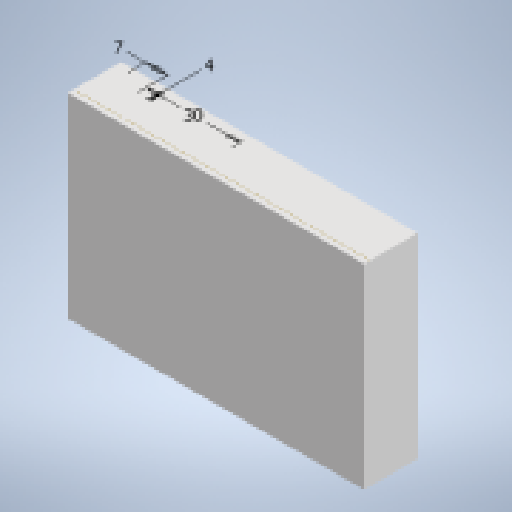
# Autodesk Inventor part: rpi4_case
Saved by Autodesk Inventor 2024 (Build 280153000, 153)
## iProperties
Created: 2024-05-03
Part Number: rpi4_case
Material: Generic
Document SubType Name: Modeling
Designer: Pintu
Density: 1 g/cm^3
Appearance: Default
Author: Pintu
Autodesk Inventor part; units mm, degrees
ref_plane "YZ Plane" through (0, 0, 0) normal (1, 0, 0) x (0, 1, 0)
ref_plane "XZ Plane" through (0, 0, 0) normal (0, 1, 0) x (-1, 0, 0)
ref_plane "XY Plane" through (0, 0, 0) normal (0, 0, 1) x (1, 0, 0)
ref_plane "Work Plane1" through (0, 0, 0) normal (0, 0, 1) x (1, 0, 0)
sketch "Sketch1" plane through (0, 0, 0) normal (0, 0, 1) x (1, 0, 0)
  line L0 (47, 31) -> (-47, 31)
  line L1 (-47, 31) -> (-47, -31)
  line L2 (-47, -31) -> (47, -31)
  line L3 (47, -31) -> (47, 31)
  line L4 (47, 31) -> (-47, -31) construction
  line L5 (-47, 31) -> (47, -31) construction
  point P0 (0, 0)
  dimension "d0" = 94
  dimension "d1" = 62
  constraints: 12 end point, 2 midpoint, 2 parallel, 1 horizontal, 1 perpendicular
  measures "d0" distance of L2.end L1.end
  measures "d1" distance of L1.end L0.end
extrude "Extrusion1" add sketch "Sketch1" along normal blind 2
sketch "Sketch2" plane through (0, 0, 0) normal (0, 0, -1) x (-1, 0, 0)
  circle A0 centre (39, 24.5) radius 3 projected
  circle A1 centre (39, 24.5) radius 1.35 projected
  circle A2 centre (39, -24.5) radius 3 projected
  circle A3 centre (39, -24.5) radius 1.35 projected
  circle A4 centre (-19, -24.5) radius 3 projected
  circle A5 centre (-19, -24.5) radius 1.35 projected
  circle A6 centre (-19, 24.5) radius 3 projected
  circle A7 centre (-19, 24.5) radius 1.35 projected
  point P0 (0, 0)
extrude "Extrusion2" add sketch "Sketch2" along normal blind 3
sketch "Sketch3" plane through (0, 0, 0) normal (0, 0, -1) x (-1, 0, 0)
  circle A0 centre (-19, -24.5) radius 3 projected
  circle A1 centre (39, -24.5) radius 3 projected
  circle A2 centre (-19, 24.5) radius 3 projected
  circle A3 centre (39, 24.5) radius 3 projected
  line L0 (47, 31) -> (47, -31) projected
  line L1 (-47, 31) -> (47, 31) projected
  line L2 (-47, -31) -> (-47, 31) projected
  line L3 (47, -31) -> (-47, -31) projected
  line L4 (45, -29) -> (45, 29)
  line L5 (45, 29) -> (-45, 29)
  line L6 (-45, 29) -> (-45, -29)
  line L7 (-45, -29) -> (45, -29)
  point P0 (0, 0)
  dimension "d6" = 2
  constraints: 8 end point, 3 other
  measures "d6" distance between parallel lines of L0 L4
extrude "Extrusion3" add sketch "Sketch3" along normal blind 15 contours L0 L3 L2 L1
sketch "Sketch4" plane through (-45, 29, 0) normal (0, -1, 0) x (1, 0, 0)
  point P0 (45, 0)
sketch "Sketch5" plane through (-45, 29, 0) normal (0, -1, 0) x (1, 0, 0)
  line L0 (0, 0) -> (90, 0) projected
  line L1 (7, 0) -> (37, 0)
  line L2 (37, 0) -> (37, -11)
  line L3 (37, -11) -> (7, -11)
  line L4 (7, -11) -> (7, 0)
  line L5 (0, 0) -> (0, -15) projected
  line L6 (90, -15) -> (0, -15) projected
  point P0 (45, 0)
  dimension "d9" = 30
  dimension "d10" = 7
  dimension "d11" = 4
  constraints: 8 end point, 2 parallel, 1 horizontal, 1 perpendicular, 1 point on line
  measures "d9" distance of L2.end L3.end
  measures "d10" distance between parallel lines of L5 L4
  measures "d11" distance between parallel lines of L6 L3
extrude "Extrusion4" cut sketch "Sketch5" against normal blind 15
body "Solid1"
